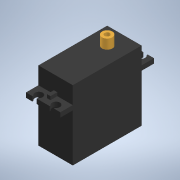
# Autodesk Inventor part: Servo
Saved by Autodesk Inventor 2020 (Build 240168000, 168)
## iProperties
Created: 2023-12-21
Part Number: Servo
Material: Generic
Document SubType Name: Modeling
Designer: smz3rm
Mass: 70 g
Surface Area: 72.7261 cm^2
Volume: 33.0719 cm^3
Density: 2.1166 g/cm^3
Appearance: Default
Author: smz3rm
Autodesk Inventor part; units mm, degrees
ref_plane "YZ Plane" through (0, 0, 0) normal (1, 0, 0) x (0, 1, 0)
ref_plane "XZ Plane" through (0, 0, 0) normal (0, 1, 0) x (-1, 0, 0)
sketch "Sketch1" plane through (0, 0, 0) normal (0, 1, 0) x (-1, 0, 0)
  line L0 (-10, 20) -> (10, 20)
  line L1 (10, 20) -> (10, -20)
  line L2 (10, -20) -> (-10, -20)
  line L3 (-10, -20) -> (-10, 20)
  line L4 (-10, 20) -> (10, -20) construction
  line L5 (10, 20) -> (-10, -20) construction
  point P0 (0, 0)
  dimension "d0" = 20
  dimension "d1" = 40
  constraints: 12 end point, 2 midpoint, 2 parallel, 1 horizontal, 1 perpendicular
  measures "d0" distance of L1.end L2.end
  measures "d1" distance of L0.end L1.end
extrude "Extrusion1" add sketch "Sketch1" along normal blind 27.7
ref_plane "Work Plane1" through (0, 27.7, 0) normal (0, 1, 0) x (1, 0, 0)
sketch "Sketch2" plane through (0, 27.7, 0) normal (0, 1, 0) x (1, 0, 0)
  line L0 (-10, 20) -> (-10, -20) projected
  line L1 (-10, -20) -> (10, -20) projected
  line L2 (10, -20) -> (10, 20) projected
  line L3 (10, 20) -> (-10, 20) projected
  point P0 (0, 0)
extrude "Extrusion2" add sketch "Sketch2" along normal blind 12.7
sketch "Sketch3" plane through (0, 27.7, 0) normal (0, 1, 0) x (1, 0, 0)
  line L0 (10, -20) -> (10, 20) projected
  line L1 (10, 20) -> (-10, 20) projected
  line L2 (-10, 20) -> (-10, -20) projected
  line L3 (-10, -20) -> (10, -20) projected
  line L4 (10, -20) -> (-10, -20)
  line L5 (-10, -20) -> (-10, -27.25)
  line L6 (-10, -27.25) -> (10, -27.25)
  line L7 (10, -27.25) -> (10, -20)
  line L8 (10, 20) -> (-10, 20)
  line L9 (-10, 20) -> (-10, 27.25)
  line L10 (-10, 27.25) -> (10, 27.25)
  line L11 (10, 27.25) -> (10, 20)
  circle A0 centre (-5, -24.75) radius 2.25
  line L12 (-14, 0) -> (14, 0) projected
  line L13 (0, 38.15) -> (0, -38.15) projected
  circle A1 centre (-5, 24.75) radius 2.25
  circle A2 centre (5, -24.75) radius 2.25
  circle A3 centre (5, 24.75) radius 2.25
  line L14 (-6.25, -27.25) -> (-6.25, -26.6208)
  line L15 (-5, -27.25) -> (-5, -27)
  line L16 (-3.75, -27.25) -> (-3.75, -26.6208)
  line L17 (-6.25, 27.25) -> (-6.25, 26.6208)
  line L18 (-3.75, 27.25) -> (-3.75, 26.6208)
  line L19 (6.25, -27.25) -> (6.25, -26.6208)
  line L20 (3.75, -27.25) -> (3.75, -26.6208)
  line L21 (6.25, 27.25) -> (6.25, 26.6208)
  line L22 (3.75, 27.25) -> (3.75, 26.6208)
  point P0 (0, 0)
  point P1 (5.7141, 27.25)
  point P2 (4.2859, 27.25)
  point P3 (-4.2859, 27.25)
  point P4 (-5.7141, 27.25)
  point P5 (-5.7141, -27.25)
  point P6 (-4.2859, -27.25)
  point P7 (4.2859, -27.25)
  point P8 (5.7141, -27.25)
  point P9 (3.75, -26.6208)
  point P10 (6.25, 26.6208)
  point P11 (-6.25, 26.6208)
  dimension "d7" = 54.5
  dimension "d8" = 10
  dimension "d9" = 49.5
  dimension "d10" = 4.5
  dimension "d13" = 2.5
  constraints: 34 end point, 17 symmetric about line, 5 collinear, 4 centre point, 4 parallel, 3 point on line, 2 horizontal, 2 perpendicular, 2 point on circle, 2 vertical, 3 other
  measures "d7" distance between parallel lines of L10 L6
  measures "d8" distance of A2.centre A0.centre
  measures "d9" distance of A1.centre A0.centre
  measures "d10" diameter of A0
  measures "d13" distance between parallel lines of L16 L14
extrude "Extrusion3" add sketch "Sketch3" along normal blind 2.7 contours L7 L6 L19 A2 L20 L13 L3 | L13 L6 L16 A0 L14 L5 L3 | L1 L13 L10 L22 A3 L21 L11 | L1 L9 L10 L17 A1 L18 L13
sketch "Sketch4" plane through (0, 30.4, 0) normal (0, 1, 0) x (1, 0, 0)
  line L0 (-10, -20) -> (10, -20) projected
  line L1 (1, -24) -> (-1, -24)
  line L2 (-1, -24) -> (-1, -20)
  line L3 (-1, -20) -> (1, -20)
  line L4 (1, -20) -> (1, -24)
  line L5 (1, -24) -> (-1, -20) construction
  line L6 (-1, -24) -> (1, -20) construction
  line L7 (0, 38.15) -> (0, -38.15) projected
  line L8 (-14, 0) -> (14, 0) projected
  line L9 (1, 24) -> (-1, 24)
  line L10 (-1, 24) -> (-1, 20)
  line L11 (1, 20) -> (1, 24)
  line L12 (-1, 20) -> (1, 20)
  line L13 (10, 20) -> (-10, 20) projected
  point P0 (0, 0)
  point P1 (0, -22)
  point P2 (0, -22)
  point P3 (1, -20)
  dimension "d14" = 2
  dimension "d15" = 4
  constraints: 20 end point, 4 symmetric about line, 3 midpoint, 2 parallel, 2 point on line, 1 collinear, 1 horizontal, 1 perpendicular
  measures "d14" distance of L1.start L1.end
  measures "d15" distance of L1.end L2.end
extrude "Extrusion4" add sketch "Sketch4" along normal blind 2
sketch "Sketch5" plane through (0, 40.4, 0) normal (0, 1, 0) x (1, 0, 0)
  circle A0 centre (0, 10) radius 3
  line L0 (10, -20) -> (10, 20) projected
  line L1 (10, 20) -> (-10, 20) projected
  line L2 (-10, 20) -> (-10, -20) projected
  line L3 (-10, -20) -> (10, -20) projected
  point P0 (0, 0)
  dimension "d18" = 6
  dimension "d19" = 30
  constraints: 1 centre point
  measures "d18" diameter of A0
  measures "d19" distance from line of L3 A0.centre
extrude "Extrusion5" add sketch "Sketch5" along normal blind 5.6 contours A0
sketch "Sketch6" plane through (0, 46, -10) normal (0, 1, 0) x (1, 0, 0)
  circle A0 centre (0, 0) radius 3 projected
  circle A1 centre (0, 0) radius 1.5
  point P0 (0, -10)
  dimension "d22" = 3
  constraints: 1 centre point, 1 coincident
  measures "d22" diameter of A1
extrude "Extrusion6" cut sketch "Sketch6" against normal up to surface (5.6 mm away) contours A1
sketch "Sketch7" plane through (10, 0, -20) normal (0, 0, -1) x (-1, 0, 0)
  line L0 (6.8, 8) -> (13.2, 8)
  line L1 (13.2, 8) -> (13.2, 4)
  line L2 (13.2, 4) -> (6.8, 4)
  line L3 (6.8, 4) -> (6.8, 8)
  line L4 (6.8, 8) -> (13.2, 4) construction
  line L5 (13.2, 8) -> (6.8, 4) construction
  line L6 (0, 0) -> (20, 0) projected
  line L7 (10, 0) -> (10, 6)
  dimension "d25" = 6.4
  dimension "d26" = 4
  dimension "d27" = 8
  constraints: 14 end point, 2 midpoint, 2 parallel, 1 horizontal, 1 perpendicular, 1 vertical
  measures "d25" distance of L1.end L2.end
  measures "d26" distance of L0.end L1.end
  measures "d27" distance between parallel lines of L6 L0
extrude "Extrusion7" add sketch "Sketch7" along normal blind 6
body "Solid1"
